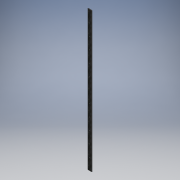
# Autodesk Inventor part: 2570 STEEL PLATE RAIL
Saved by Autodesk Inventor 2018 (Build 220112000, 112)
## iProperties
Created: 2018-10-15
Part Number: 2570 STEEL PLATE RAIL
Material: Acero
Document SubType Name: Modeling
Designer: Toshiba
Density: 7.85 g/cm^3
Appearance: Placa
Author: Toshiba
Autodesk Inventor part; units mm, degrees
ref_plane "YZ Plane" through (0, 0, 0) normal (1, 0, 0) x (0, 1, 0)
ref_plane "XZ Plane" through (0, 0, 0) normal (0, 1, 0) x (-1, 0, 0)
ref_plane "XY Plane" through (0, 0, 0) normal (0, 0, 1) x (1, 0, 0)
sketch "Boceto1" plane through (0, 0, 0) normal (0, 1, 0) x (-1, 0, 0)
  line L0 (-37.5, -1285) -> (-37.5, 1285)
  line L1 (-37.5, 1285) -> (37.5, 1285)
  line L2 (37.5, 1285) -> (37.5, -1285)
  line L3 (37.5, -1285) -> (-37.5, -1285)
  line L4 (-37.5, -1285) -> (37.5, 1285) construction
  line L5 (-37.5, 1285) -> (37.5, -1285) construction
  point P0 (0, 0)
  dimension "d0" = 2570
  dimension "d1" = 75
  constraints: 12 end point, 2 midpoint, 2 parallel, 1 perpendicular, 1 vertical
  measures "d0" distance of L0.start L0.end
  measures "d1" distance of L0.end L1.end
extrude "Extrusión1" add sketch "Boceto1" along normal blind 10
sketch "Boceto2" plane through (0, 10, 0) normal (0, 1, 0) x (1, 0, 0)
  circle A0 centre (0, -1071) radius 5
  line L0 (20, -1285) -> (-20, -1285)
  circle A1 centre (0, -857) radius 5
  circle A2 centre (0, -643) radius 5
  circle A3 centre (0, -429) radius 5
  circle A4 centre (0, -215) radius 5
  line L1 (-157.4788, 0) -> (166.1246, 0)
  circle A5 centre (0, 1071) radius 5
  circle A6 centre (0, 857) radius 5
  circle A7 centre (0, 643) radius 5
  circle A8 centre (0, 429) radius 5
  circle A9 centre (0, 215) radius 5
  point P0 (0, 0)
  point P1 (0, 0)
  dimension "d4" = 10
  dimension "d5" = 214
  dimension "d6" = 10
  dimension "d7" = 214
  dimension "d8" = 10
  dimension "d9" = 214
  dimension "d10" = 10
  dimension "d11" = 214
  dimension "d12" = 10
  dimension "d13" = 214
  dimension "d14" = 215
  constraints: 10 centre point, 5 symmetric about line, 4 end point, 1 horizontal, 5 other
  measures "d4" diameter of A0
  measures "d5" distance from line of L0 A0.centre
  measures "d6" diameter of A1
  measures "d7" distance of A0.centre A1.centre
  measures "d8" diameter of A2
  measures "d9" distance of A1.centre A2.centre
  measures "d10" diameter of A3
  measures "d11" distance of A2.centre A3.centre
  measures "d12" diameter of A4
  measures "d13" distance of A3.centre A4.centre
  measures "d14" distance from line of L1 A4.centre
extrude "Extrusión2" cut sketch "Boceto2" against normal blind 10
